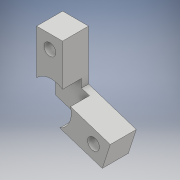
# Autodesk Inventor part: 鸦片下
Saved by Autodesk Inventor 2018 (Build 220112000, 112)
## iProperties
Created: 2021-03-02
Part Number: 鸦片下
Material: 常规
Document SubType Name: Modeling
Designer: OHHHHHHHHHH
Density: 1 g/cm^3
Appearance: 默认
Author: OHHHHHHHHHH
## iProperties of the stored document 压片下666_3D 打印.ipt
Created: 2021-03-03
Part Number: 压片下666_3D 打印
Material: 常规
Document SubType Name: Modeling
Designer: OHHHHHHHHHH
Density: 1 g/cm^3
Appearance: 默认
Author: OHHHHHHHHHH
Autodesk Inventor part; units mm, degrees
ref_plane "YZ Plane" through (0, 0, 0) normal (1, 0, 0) x (0, 1, 0)
ref_plane "XZ Plane" through (0, 0, 0) normal (0, 1, 0) x (-1, 0, 0)
ref_plane "XY Plane" through (0, 0, 0) normal (0, 0, 1) x (1, 0, 0)
sketch "草图1" plane through (0, 0, 0) normal (0, 1, 0) x (-1, 0, 0)
  circle A0 centre (-11.3094, -1.4762) radius 1.25
  circle A1 centre (-2.0908, 11.2121) radius 1.25
  line L0 (-5.7974, 4.2121) -> (1.6092, -1.1691) construction
  line L1 (0.7195, 14.068) -> (0.7195, -0.5227)
  line L2 (-4.7634, 3.4608) -> (-4.7634, 14.068)
  line L3 (-4.7634, 14.068) -> (0.7195, 14.068)
  line L4 (-4.7634, 3.4608) -> (-14.8514, 0.183)
  line L5 (-14.8514, 0.183) -> (-13.1571, -5.0315)
  line L6 (-13.1571, -5.0315) -> (0.7195, -0.5227)
  point P0 (0, 0)
  dimension "d0" = 2.5
  constraints: 14 end point, 3 symmetric about line, 2 centre point, 2 point on line, 2 vertical, 1 perpendicular, 1 other
  measures "d0" diameter of A1
extrude "拉伸1" add sketch "草图1" along normal blind 5.5
sketch "草图3" plane through (0, 0, 0) normal (0, -1, 0) x (1, 0, 0)
  line L0 (-0.7195, -0.5227) -> (-0.7195, 14.068) construction
  line L1 (4.7634, 14.068) -> (4.7634, 3.4608) construction
  line L2 (-0.7195, -0.5227) -> (4.7634, 3.4608) construction
  circle A0 centre (2.0908, 11.2121) radius 1.25 construction
  circle A1 centre (11.3094, -1.4762) radius 1.25 construction
  line L3 (-0.7195, -0.5227) -> (-0.7195, 14.068) construction
  line L4 (13.1571, -5.0315) -> (-0.7195, -0.5227) construction
  line L5 (14.8514, 0.183) -> (13.1571, -5.0315) construction
  line L6 (4.7634, 3.4608) -> (14.8514, 0.183) construction
  line L7 (4.7634, 14.068) -> (4.7634, 3.4608) construction
  line L8 (-0.7195, 14.068) -> (4.7634, 14.068) construction
  circle A2 centre (2.3678, 1.7203) radius 4.25
  point P0 (0, 0)
  dimension "d7" = 8.5
  constraints: 2 end point, 1 centre point, 1 point on line
  measures "d7" diameter of A2
extrude "拉伸2" cut sketch "草图3" against normal blind 4
sketch "草图5" plane through (0, 5.5, 0) normal (0, 1, 0) x (1, 0, 0)
  line L0 (-0.7195, 0.5227) -> (4.7634, -3.4608)
  line L1 (0.7578, -0.5506) -> (0.7578, -7.5215)
  line L2 (0.7578, -7.5215) -> (3.7578, -7.5215)
  line L3 (3.7578, -7.5215) -> (3.7578, -2.7302)
  line L4 (0.7578, -0.5506) -> (7.3875, 1.6036)
  line L5 (7.3875, 1.6036) -> (8.3146, -1.2496)
  line L6 (8.3146, -1.2496) -> (3.7578, -2.7302)
  circle A0 centre (2.0908, -11.2121) radius 1.25 construction
  point P0 (0, 0)
  dimension "d15" = 7.3812
  constraints: 14 end point, 2 perpendicular, 2 point on line, 2 symmetric about line, 1 vertical
  measures "d15" diameter of A0.centre L2
extrude "拉伸3" add sketch "草图5" along normal blind 1.5
chamfer "倒角1" distance 1 angle 45 6 edges at (2.2578, 7, 7.5215) (3.7578, 7, 5.1258) (6.0362, 7, 1.9899) (7.851, 7, -0.177) (4.0727, 7, -0.5265) (0.7578, 7, 4.036)
sketch "草图6" plane through (0, 5.5, 0) normal (0, 1, 0) x (1, 0, 0)
  point P0 (0, 0)
